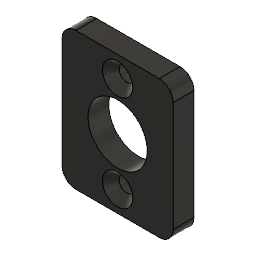
magstrap (Autodesk Fusion 360 archive; units mm, degrees)
design "UHMW Spacer"
Autodesk Fusion 360 part; units mm, degrees
sketch "Sketch1" plane through (0, 0, 38.1) normal (0, 0, 1) x (0, 1, 0)
  circle A0 centre (0, -127) radius 13.5
  circle A1 centre (0, -76.2) radius 13.5
  circle A2 centre (0, -25.4) radius 13.5
  circle A3 centre (0, 76.2) radius 13.5
  circle A4 centre (0, 127) radius 13.5
  line L0 (34.29, -152.4) -> (34.29, 152.4)
  line L1 (34.29, 152.4) -> (-34.29, 152.4)
  line L2 (-34.29, 152.4) -> (-34.29, -152.4)
  line L3 (-34.29, -152.4) -> (34.29, -152.4)
  line L4 (-25.0825, 50.8) -> (25.0825, 50.8)
  line L5 (31.4325, 44.45) -> (31.4325, 6.35)
  line L6 (25.0825, 0) -> (-25.0825, 0)
  line L7 (-31.4325, 6.35) -> (-31.4325, 44.45)
  line L8 (-31.4325, -152.4) -> (-31.4325, 152.4)
  line L9 (31.4325, -152.4) -> (31.4325, 152.4)
  arc A5 (-25.0825, 50.8) -> (-31.4325, 44.45) centre (-25.0825, 44.45) ccw
  arc A6 (-31.4325, 6.35) -> (-25.0825, 0) centre (-25.0825, 6.35) ccw
  arc A7 (25.0825, 0) -> (31.4325, 6.35) centre (25.0825, 6.35) ccw
  arc A8 (31.4325, 44.45) -> (25.0825, 50.8) centre (25.0825, 44.45) ccw
  circle A9 centre (0, 25.4) radius 13.5
  circle A10 centre (0, 25.4) radius 13.5
  dimension "d45" = 6.35
  dimension "d47" = 62.865
  dimension "d313" = 27
  dimension "d314" = 25.4
  dimension "d315" = 31.4325
  dimension "d316" = 25.4
  constraint horizontal L4
  constraint vertical L5
  constraint horizontal L6
  constraint vertical L7
  constraint tangent L4 A5
  constraint tangent L7 A5
  constraint tangent L6 A6
  constraint tangent L7 A6
  constraint equal A5 A6
  constraint tangent L5 A7
  constraint tangent L6 A7
  constraint equal A5 A7
  constraint tangent L4 A8
  constraint tangent L5 A8
  constraint equal A5 A8
  constraint concentric A9 A10
  measures "d45" radius of A5
  measures "d47" distance of L5 L7
  measures "d313" diameter of A9
  measures "d314" distance of L4 A9.centre
  measures "d315" distance of L7 A9.centre
  measures "d316" distance of L6 A9.centre
extrude "Extrude1" add sketch "Sketch1" along normal blind 9.525 contours L4 L5 L6 L7 L8 L9 A5 A6 A7 A8
sketch "Sketch2" plane through (0, 0, 47.625) normal (0, 0, 1) x (1, 0, 0)
  circle A0 centre (-25.4, 0) radius 13.5
  arc A1 (0, 25.0825) -> (-6.35, 31.4325) centre (-6.35, 25.0825) ccw
  line L0 (-6.35, 31.4325) -> (-44.45, 31.4325)
  arc A2 (-44.45, 31.4325) -> (-50.8, 25.0825) centre (-44.45, 25.0825) ccw
  line L1 (-50.8, 25.0825) -> (-50.8, -25.0825)
  arc A3 (-50.8, -25.0825) -> (-44.45, -31.4325) centre (-44.45, -25.0825) ccw
  line L2 (-44.45, -31.4325) -> (-6.35, -31.4325)
  arc A4 (-6.35, -31.4325) -> (0, -25.0825) centre (-6.35, -25.0825) ccw
  line L3 (0, -25.0825) -> (0, 25.0825)
  line L4 (0, 0) -> (-50.8, 0) construction
  point P0 (-25.4, 21.9075)
  point P1 (-25.4, -21.9075)
  dimension "d1" = 9.525
  dimension "d2" = 25.4
  constraint coincident L4.start origin
  constraint midpoint L1 L4.end
  constraint symmetric P0 P1 L4
  measures "d1" distance of L0 P0
  measures "d2" distance of L3 P0
hole "Hole10" at (-25.4, 21.9075, 47.625) at (-25.4, -21.9075, 47.625) direction (0, 0, -1) diameter 6.7564 end through all countersink diameter 13.843 countersink angle 82
equation "d313 = upright_hole_dia"
equation "upright_hole_dia = 27 mm"
